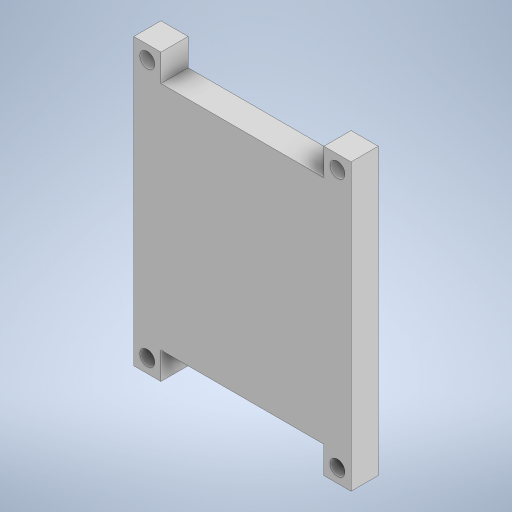
# Autodesk Inventor part: battery_box_cap_ver2
Saved by Autodesk Inventor 2023 (Build 270158000, 158)
## iProperties
Created: 2023-05-21
Part Number: battery_box_cap_ver2
Material: 一般
Document SubType Name: Modeling
Designer: 310611102
Density: 1 g/cm^3
Appearance: 預設
Author: 310611102
Autodesk Inventor part; units mm, degrees
ref_plane "YZ Plane" through (0, 0, 0) normal (1, 0, 0) x (0, 1, 0)
ref_plane "XZ Plane" through (0, 0, 0) normal (0, 1, 0) x (-1, 0, 0)
ref_plane "XY Plane" through (0, 0, 0) normal (0, 0, 1) x (1, 0, 0)
sketch "Sketch1" plane through (0, 0, 0) normal (0, 0, 1) x (1, 0, 0)
  line L0 (-40, 42.5) -> (40, 42.5)
  line L1 (40, 42.5) -> (40, -42.5)
  line L2 (40, -42.5) -> (-40, -42.5)
  line L3 (-40, -42.5) -> (-40, 42.5)
  line L4 (-40, 42.5) -> (40, -42.5) construction
  line L5 (40, 42.5) -> (-40, -42.5) construction
  line L6 (40, 42.5) -> (30, 42.5)
  line L7 (30, 42.5) -> (30, 52.5)
  line L8 (30, 52.5) -> (40, 52.5)
  line L9 (40, 52.5) -> (40, 42.5)
  line L10 (-40, 42.5) -> (-30, 42.5)
  line L11 (-30, 42.5) -> (-30, 52.5)
  line L12 (-30, 52.5) -> (-40, 52.5)
  line L13 (-40, 52.5) -> (-40, 42.5)
  line L14 (-40, -42.5) -> (-30, -42.5)
  line L15 (-30, -42.5) -> (-30, -52.5)
  line L16 (-30, -52.5) -> (-40, -52.5)
  line L17 (-40, -52.5) -> (-40, -42.5)
  line L18 (40, -42.5) -> (30, -42.5)
  line L19 (30, -42.5) -> (30, -52.5)
  line L20 (30, -52.5) -> (40, -52.5)
  line L21 (40, -52.5) -> (40, -42.5)
  circle A0 centre (-35, 47.5) radius 2.75
  circle A1 centre (35, 47.5) radius 2.75
  circle A2 centre (35, -47.5) radius 2.75
  circle A3 centre (-35, -47.5) radius 2.75
  point P0 (0, 0)
  point P1 (-35, 52.5)
  point P2 (35, 52.5)
  point P3 (-40, -47.5)
  point P4 (-40, 47.5)
  point P5 (30, -42.5)
  point P6 (30, 42.5)
  point P7 (30, -47.5)
  dimension "d1" = 10
  dimension "d2" = 10
  dimension "d3" = 5.5
  dimension "d4" = 5.5
  dimension "d5" = 5.5
  dimension "d6" = 5.5
  dimension "d7" = 10
  dimension "d8" = 10
  dimension "d9" = 85
  dimension "d10" = 80
  constraints: 44 end point, 10 parallel, 7 midpoint, 5 horizontal, 5 perpendicular, 4 centre point, 4 horizontal alignment, 4 vertical alignment, 3 point on line, 1 collinear
  measures "d1" distance of L11.end L12.end
  measures "d2" distance of L12.end L0.start
  measures "d3" diameter of A0
  measures "d4" diameter of A1
  measures "d5" diameter of A2
  measures "d6" diameter of A3
  measures "d7" distance of L16.end L2.end
  measures "d8" distance of L7.end L8.end
  measures "d9" distance between parallel lines of L2 L0
  measures "d10" distance of L0.start L0.end
extrude "Extrusion1" add sketch "Sketch1" along normal blind 10
body "Solid1"
